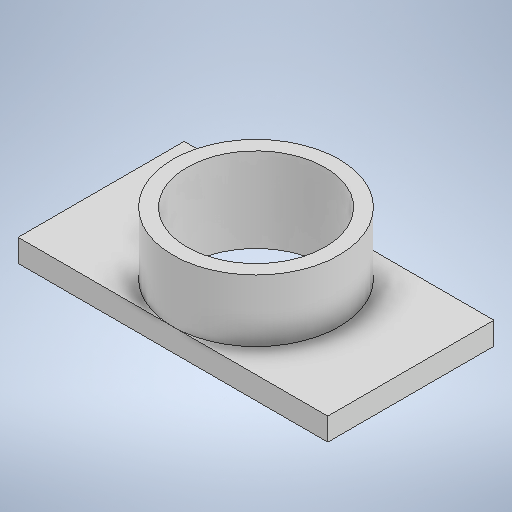
# Autodesk Inventor part: mic-mic-holder
Saved by Autodesk Inventor 2025.2 (Build 292293000, 293)
## iProperties
Created: 2025-04-19
Part Number: mic-mic-holder
Material: Generic
Document SubType Name: Modeling
Designer: tdeboutte
Density: 1 g/cm^3
Appearance: Default
Author: tdeboutte
Autodesk Inventor part; units mm, degrees
ref_plane "YZ Plane" through (0, 0, 0) normal (1, 0, 0) x (0, 1, 0)
ref_plane "XZ Plane" through (0, 0, 0) normal (0, 1, 0) x (-1, 0, 0)
ref_plane "XY Plane" through (0, 0, 0) normal (0, 0, 1) x (1, 0, 0)
sketch "Sketch1" plane through (0, 0, 0) normal (0, 1, 0) x (-1, 0, 0)
  circle A0 centre (0, 0) radius 4.9
  circle A1 centre (0, 0) radius 5.9
  dimension "d0" = 9.8
  dimension "d1" = 1
  constraints: 2 centre point, 1 coincident
  measures "d0" diameter of A0
  measures "d1" radial gap between concentric circles of A0 A1
extrude "Extrusion1" add sketch "Sketch1" along normal blind 6
sketch "Sketch2" plane through (0, 0, 0) normal (0, -1, 0) x (1, 0, 0)
  circle A0 centre (0, 0) radius 5.9 projected
  circle A1 centre (0, 0) radius 4.9 projected
  line L0 (-11, 5.9) -> (11, 5.9)
  line L1 (11, 5.9) -> (11, -5.9)
  line L2 (11, -5.9) -> (-11, -5.9)
  line L3 (-11, -5.9) -> (-11, 5.9)
  line L4 (-11, 5.9) -> (11, -5.9) construction
  line L5 (11, 5.9) -> (-11, -5.9) construction
  circle A2 centre (0, 0) radius 5.9 projected
  point P0 (0, -5.9)
  point P1 (0, 5.9)
  dimension "d4" = 22
  constraints: 12 end point, 2 midpoint, 2 parallel, 2 tangent, 1 horizontal, 1 perpendicular
  measures "d4" distance of L1.end L2.end
extrude "Extrusion2" add sketch "Sketch2" against normal blind 1.6 contours A0 L0 L1 L2 | A0 L2 L3 L0
body "Solid1"
